Autodesk Fusion 360 part; units mm, degrees
(part 3 of 3)
  line L1749 (208.3944, 281.0774) -> (206.5826, 280.7265)
  line L1750 (222.9841, 283.0826) -> (221.6889, 282.9561)
  line L1751 (248.9543, 186.6306) -> (249.0021, 186.3543)
  line L1752 (195.2165, 277.6676) -> (195.1345, 277.5743)
  line L1753 (282.2262, 282.3149) -> (280.3205, 282.5523)
  line L1754 (274.0771, 283.1906) -> (271.0467, 283.4676)
  line L1755 (195.1011, 277.4923) -> (198.2479, 273.2051)
  line L1756 (284.0442, 282.0682) -> (282.2262, 282.3149)
  line L1757 (206.5826, 280.7265) -> (204.8864, 280.373)
  line L1758 (212.3645, 281.7592) -> (210.3217, 281.4227)
  line L1759 (195.3395, 277.767) -> (195.2165, 277.6676)
  line L1760 (229.8917, 283.6109) -> (228.4526, 283.5204)
  line L1761 (249.0554, 186.0895) -> (249.1147, 185.8662)
  line L1762 (249.0021, 186.3543) -> (249.0554, 186.0895)
  line L1763 (276.246, 282.992) -> (274.0771, 283.1906)
  line L1764 (291.8211, 280.761) -> (290.4407, 281.0262)
  line L1765 (297.4131, 279.4996) -> (296.4692, 279.7372)
  line L1766 (299.3168, 278.9841) -> (298.2698, 279.2731)
  line L1767 (195.1345, 277.5743) -> (195.1112, 277.5316)
  line L1768 (221.6889, 282.9561) -> (220.4225, 282.8236)
  line L1769 (274.6565, 267.6572) -> (275.3635, 267.5207)
  line L1770 (291.1421, 264.0873) -> (291.6993, 264.4176)
  line L1771 (264.1428, 259.2261) -> (264.6603, 261.8646)
  line L1772 (284.4844, 260.9375) -> (284.5965, 260.9561)
  line L1773 (266.1501, 268.214) -> (266.1932, 268.2563)
  line L1774 (279.5002, 266.3305) -> (280.0419, 266.1024)
  line L1775 (278.9516, 266.543) -> (279.5002, 266.3305)
  line L1776 (248.8733, 187.0975) -> (248.9543, 186.6306)
  line L1777 (281.7836, 265.2546) -> (283.7059, 263.1269)
  line L1778 (266.0031, 267.9084) -> (266.0551, 268.04)
  line L1779 (249.2535, 185.6642) -> (249.2927, 185.6866)
  line L1780 (285.7031, 261.3881) -> (286.7992, 261.8821)
  line L1781 (249.1147, 185.8662) -> (249.1468, 185.7794)
  line L1782 (249.2161, 185.6747) -> (249.2345, 185.6656)
  line L1783 (280.8861, 265.7216) -> (281.1981, 265.5867)
  line L1784 (266.1041, 268.1418) -> (266.1501, 268.214)
  line L1785 (277.2718, 267.0843) -> (277.8367, 266.9201)
  line L1786 (280.5762, 265.859) -> (280.8861, 265.7216)
  line L1787 (266.0551, 268.04) -> (266.1041, 268.1418)
  line L1788 (284.3283, 260.9546) -> (284.3773, 260.9402)
  line L1789 (272.8993, 267.9499) -> (273.424, 267.8705)
  line L1790 (272.4361, 268.0131) -> (272.8993, 267.9499)
  line L1791 (265.762, 267.0883) -> (265.8894, 267.557)
  line L1792 (290.0115, 263.4568) -> (290.5793, 263.7671)
  line L1793 (290.5793, 263.7671) -> (291.1421, 264.0873)
  line L1794 (288.8641, 262.8646) -> (289.4395, 263.1561)
  line L1795 (265.4627, 265.8028) -> (265.6201, 266.5033)
  line L1796 (265.6201, 266.5033) -> (265.762, 267.0883)
  line L1797 (249.1806, 185.7144) -> (249.2161, 185.6747)
  line L1798 (284.2839, 260.9802) -> (284.3283, 260.9546)
  line L1799 (284.8032, 261.0126) -> (285.003, 261.0906)
  line L1800 (283.7059, 263.1269) -> (284.2839, 260.9802)
  line L1801 (281.3514, 265.5148) -> (281.501, 265.4369)
  line L1802 (265.0979, 264.0592) -> (265.4627, 265.8028)
  line L1803 (249.3339, 185.7457) -> (258.622, 231.7438)
  line L1804 (281.1981, 265.5867) -> (281.3514, 265.5148)
  line L1805 (249.2345, 185.6656) -> (249.2535, 185.6642)
  line L1806 (288.2859, 262.5822) -> (288.8641, 262.8646)
  line L1807 (281.6455, 265.3509) -> (281.7836, 265.2546)
  line L1808 (265.8894, 267.557) -> (266.0031, 267.9084)
  line L1809 (289.4395, 263.1561) -> (290.0115, 263.4568)
  line L1810 (275.3635, 267.5207) -> (276.1304, 267.3625)
  line L1811 (278.3969, 266.7396) -> (278.9516, 266.543)
  line L1812 (262.8388, 252.6458) -> (264.1428, 259.2261)
  line L1813 (284.7044, 260.9802) -> (284.8032, 261.0126)
  line L1814 (276.7028, 267.2318) -> (277.2718, 267.0843)
  line L1815 (274.0099, 267.7734) -> (274.6565, 267.6572)
  line L1816 (277.8367, 266.9201) -> (278.3969, 266.7396)
  line L1817 (273.424, 267.8705) -> (274.0099, 267.7734)
  line L1818 (284.5965, 260.9561) -> (284.7044, 260.9802)
  line L1819 (285.003, 261.0906) -> (285.7031, 261.3881)
  line L1820 (266.1932, 268.2563) -> (271.6958, 268.0958)
  line L1821 (291.6993, 264.4176) -> (292.2502, 264.7585)
  line L1822 (264.6603, 261.8646) -> (265.0979, 264.0592)
  line L1823 (280.0419, 266.1024) -> (280.5762, 265.859)
  line L1824 (284.3773, 260.9402) -> (284.4844, 260.9375)
  line L1825 (271.6958, 268.0958) -> (272.4361, 268.0131)
  line L1826 (258.622, 231.7438) -> (262.8388, 252.6458)
  line L1827 (292.2502, 264.7585) -> (292.7939, 265.11)
  line L1828 (286.7992, 261.8821) -> (288.2859, 262.5822)
  line L1829 (292.7939, 265.11) -> (293.3298, 265.4726)
  line L1830 (249.2927, 185.6866) -> (249.3339, 185.7457)
  line L1831 (276.1304, 267.3625) -> (276.7028, 267.2318)
  line L1832 (281.501, 265.4369) -> (281.6455, 265.3509)
  line L1833 (296.8008, 268.3446) -> (297.5669, 269.108)
  line L1834 (256.4399, 274.4982) -> (255.4396, 274.4952)
  line L1835 (294.8833, 266.6296) -> (295.3806, 267.0393)
  line L1836 (294.1268, 270.7552) -> (293.2879, 270.975)
  line L1837 (225.7816, 274.1169) -> (224.6982, 274.023)
  line L1838 (294.7936, 270.5692) -> (294.1268, 270.7552)
  line L1839 (255.1595, 274.4828) -> (255.0748, 274.4732)
  line L1840 (223.4692, 273.9056) -> (222.0948, 273.7634)
  line L1841 (293.2879, 270.975) -> (292.2757, 271.2235)
  line L1842 (295.7733, 270.2687) -> (295.2895, 270.4226)
  line L1843 (247.0886, 270.1383) -> (246.1685, 271.255)
  line L1844 (297.7654, 269.3164) -> (297.8145, 269.3775)
  line L1845 (276.8823, 273.6786) -> (275.0317, 273.8458)
  line L1846 (244.2152, 273.6532) -> (243.8236, 274.1236)
  line L1847 (243.4699, 274.5089) -> (243.4129, 274.5502)
  line L1848 (222.0948, 273.7634) -> (220.5752, 273.5951)
  line L1849 (291.089, 271.4951) -> (289.7268, 271.7846)
  line L1850 (284.2508, 272.7625) -> (282.4148, 273.0309)
  line L1851 (224.6982, 274.023) -> (223.4692, 273.9056)
  line L1852 (292.2757, 271.2235) -> (291.089, 271.4951)
  line L1853 (296.3401, 267.8965) -> (296.8008, 268.3446)
  line L1854 (246.1685, 271.255) -> (244.7346, 273.0159)
  line L1855 (275.0317, 273.8458) -> (273.1788, 273.9905)
  line L1856 (243.4129, 274.5502) -> (227.5104, 274.2394)
  line L1857 (249.1468, 185.7794) -> (249.1806, 185.7144)
  line L1858 (271.324, 274.1137) -> (269.4679, 274.2167)
  line L1859 (295.2895, 270.4226) -> (294.7936, 270.5692)
  line L1860 (322.7332, 314.692) -> (322.4298, 314.9296)
  line L1861 (323.7048, 313.8093) -> (323.3126, 314.1859)
  line L1862 (324.7886, 303.6366) -> (324.9042, 304.9171)
  line L1863 (310.0792, 323.0626) -> (308.9507, 323.6614)
  line L1864 (324.3257, 313.1815) -> (324.042, 313.474)
  line L1865 (297.9477, 328.7065) -> (296.4619, 329.2882)
  line L1866 (287.4008, 332.3961) -> (285.8705, 332.8536)
  line L1867 (320.2812, 316.2527) -> (320.1962, 316.3038)
  line L1868 (319.2981, 317.184) -> (318.947, 317.4895)
  line L1869 (324.9042, 304.9171) -> (324.9497, 305.5581)
  line L1870 (273.5972, 335.802) -> (271.5875, 336.1301)
  line L1871 (320.1155, 316.3616) -> (319.96, 316.5293)
  line L1872 (319.8006, 316.6988) -> (319.5813, 316.9188)
  line L1873 (224.4972, 335.6447) -> (223.0698, 335.3643)
  line L1874 (308.9507, 323.6614) -> (307.7593, 324.2748)
  line L1875 (259.2802, 337.7554) -> (258.6668, 337.7919)
  line L1876 (215.9614, 333.7319) -> (214.548, 333.3588)
  line L1877 (239.6725, 337.7845) -> (238.9752, 337.7305)
  line L1878 (228.8057, 336.401) -> (227.355, 336.1599)
  line L1879 (323.0278, 314.4444) -> (322.7332, 314.692)
  line L1880 (211.7322, 332.5656) -> (210.3306, 332.1453)
  line L1881 (302.3544, 326.8458) -> (300.8944, 327.4857)
  line L1882 (324.5868, 301.5321) -> (324.7886, 303.6366)
  line L1883 (210.3306, 332.1453) -> (208.9336, 331.7091)
  line L1884 (322.1188, 315.1576) -> (321.8012, 315.3769)
  line L1885 (316.2634, 319.4035) -> (315.5599, 319.859)
  line L1886 (319.96, 316.5293) -> (319.8006, 316.6988)
  line L1887 (320.8196, 315.9883) -> (320.642, 316.0799)
  line L1888 (323.3126, 314.1859) -> (323.0278, 314.4444)
  line L1889 (320.1962, 316.3038) -> (320.1155, 316.3616)
  line L1890 (313.9751, 320.843) -> (313.0927, 321.3687)
  line L1891 (318.0248, 318.2006) -> (317.4953, 318.5728)
  line L1892 (318.947, 317.4895) -> (318.5239, 317.83)
  line L1893 (315.5599, 319.859) -> (314.7973, 320.3393)
  line L1894 (320.4596, 316.1634) -> (320.2812, 316.2527)
  line L1895 (324.042, 313.474) -> (323.7048, 313.8093)
  line L1896 (321.4781, 315.588) -> (320.8196, 315.9883)
  line L1897 (314.7973, 320.3393) -> (313.9751, 320.843)
  line L1898 (217.378, 334.0893) -> (215.9614, 333.7319)
  line L1899 (299.4254, 328.1058) -> (297.9477, 328.7065)
  line L1900 (316.9084, 318.9743) -> (316.2634, 319.4035)
  line L1901 (322.4298, 314.9296) -> (322.1188, 315.1576)
  line L1902 (324.9795, 306.2) -> (324.9836, 312.4179)
  line L1903 (318.5239, 317.83) -> (318.0248, 318.2006)
  line L1904 (218.7976, 334.4312) -> (217.378, 334.0893)
  line L1905 (307.7593, 324.2748) -> (306.5046, 324.9014)
  line L1906 (324.9491, 312.4721) -> (324.8674, 312.5772)
  line L1907 (225.9257, 335.9099) -> (224.4972, 335.6447)
  line L1908 (214.548, 333.3588) -> (213.1381, 332.9701)
  line L1909 (293.4676, 330.3955) -> (291.96, 330.9219)
  line L1910 (276.8835, 335.1874) -> (276.1537, 335.3356)
  line L1911 (275.3627, 335.4875) -> (273.5972, 335.802)
  line L1912 (213.1381, 332.9701) -> (211.7322, 332.5656)
  line L1913 (324.8674, 312.5772) -> (324.5569, 312.9335)
  line L1914 (321.8012, 315.3769) -> (321.4781, 315.588)
  line L1915 (319.5813, 316.9188) -> (319.2981, 317.184)
  line L1916 (324.9497, 305.5581) -> (324.9795, 306.2)
  line L1917 (306.5046, 324.9014) -> (305.1859, 325.5398)
  line L1918 (313.0927, 321.3687) -> (312.1496, 321.9148)
  line L1919 (324.9836, 312.4179) -> (324.9491, 312.4721)
  line L1920 (320.642, 316.0799) -> (320.4596, 316.1634)
  line L1921 (324.5569, 312.9335) -> (324.3257, 313.1815)
  line L1922 (311.1453, 322.4799) -> (310.0792, 323.0626)
  line L1923 (258.6668, 337.7919) -> (240.0115, 337.8045)
  line L1924 (317.4953, 318.5728) -> (316.9084, 318.9743)
  line L1925 (305.1859, 325.5398) -> (303.8026, 326.1884)
  line L1926 (261.1143, 337.5583) -> (260.5038, 337.6319)
  line L1927 (282.7966, 333.72) -> (281.2539, 334.1295)
  line L1928 (276.1537, 335.3356) -> (275.3627, 335.4875)
  line L1929 (264.0969, 337.1857) -> (261.1143, 337.5583)
  line L1930 (237.9214, 337.6332) -> (236.5123, 337.4828)
  line L1931 (294.9684, 329.851) -> (293.4676, 330.3955)
  line L1932 (300.8944, 327.4857) -> (299.4254, 328.1058)
  line L1933 (278.1594, 334.9028) -> (277.5521, 335.0431)
  line L1934 (279.7081, 334.5236) -> (278.1594, 334.9028)
  line L1935 (288.9262, 331.9218) -> (287.4008, 332.3961)
  line L1936 (277.5521, 335.0431) -> (276.8835, 335.1874)
  line L1937 (240.0115, 337.8045) -> (239.6725, 337.7845)
  line L1938 (200.6691, 328.7549) -> (199.3146, 328.2058)
  line L1939 (177.1697, 315.6333) -> (176.7433, 315.3633)
  line L1940 (284.3356, 333.2948) -> (282.7966, 333.72)
  line L1941 (173.7111, 312.2406) -> (173.6926, 312.1123)
  line L1942 (266.837, 336.8229) -> (264.0969, 337.1857)
  line L1943 (227.355, 336.1599) -> (225.9257, 335.9099)
  line L1944 (312.1496, 321.9148) -> (311.1453, 322.4799)
  line L1945 (259.8925, 337.6999) -> (259.2802, 337.7554)
  line L1946 (199.3146, 328.2058) -> (197.9676, 327.6402)
  line L1947 (197.9676, 327.6402) -> (196.6284, 327.0581)
  line L1948 (269.3339, 336.4707) -> (266.837, 336.8229)
  line L1949 (271.5875, 336.1301) -> (269.3339, 336.4707)
  line L1950 (290.446, 331.4305) -> (288.9262, 331.9218)
  line L1951 (223.0698, 335.3643) -> (221.6438, 335.0687)
  line L1952 (181.7405, 319.0373) -> (180.9539, 318.5041)
  line L1953 (230.1694, 336.618) -> (228.8057, 336.401)
  line L1954 (260.5038, 337.6319) -> (259.8925, 337.6999)
  line L1955 (236.5123, 337.4828) -> (234.7496, 337.2699)
  line L1956 (177.8228, 316.0135) -> (177.6023, 315.892)
  line L1957 (175.565, 314.5732) -> (175.3879, 314.4285)
  line L1958 (234.7496, 337.2699) -> (233.7361, 337.1369)
  line L1959 (206.155, 330.7888) -> (204.7741, 330.3046)
  line L1960 (296.4619, 329.2882) -> (294.9684, 329.851)
  line L1961 (191.3572, 324.5639) -> (190.0625, 323.8985)
  line L1962 (202.0308, 329.2877) -> (200.6691, 328.7549)
  line L1963 (285.8705, 332.8536) -> (284.3356, 333.2948)
  line L1964 (233.7361, 337.1369) -> (232.6348, 336.9848)
  line L1965 (178.0471, 316.128) -> (177.8228, 316.0135)
  line L1966 (173.6724, 310.891) -> (173.687, 310.2069)
  line L1967 (220.2196, 334.7577) -> (218.7976, 334.4312)
  line L1968 (232.6348, 336.9848) -> (231.4459, 336.8122)
  line L1969 (221.6438, 335.0687) -> (220.2196, 334.7577)
  line L1970 (303.8026, 326.1884) -> (302.3544, 326.8458)
  line L1971 (175.2175, 314.2767) -> (175.0547, 314.1173)
  line L1972 (231.4459, 336.8122) -> (230.1694, 336.618)
  line L1973 (238.9752, 337.7305) -> (237.9214, 337.6332)
  line L1974 (203.3992, 329.8043) -> (202.0308, 329.2877)
  line L1975 (190.0625, 323.8985) -> (188.7779, 323.2162)
  line L1976 (175.9345, 314.8439) -> (175.7475, 314.7115)
  line L1977 (175.3879, 314.4285) -> (175.2175, 314.2767)
  line L1978 (291.96, 330.9219) -> (290.446, 331.4305)
  line L1979 (281.2539, 334.1295) -> (279.7081, 334.5236)
  line L1980 (178.3376, 316.3185) -> (178.1982, 316.2147)
extrude "Extrude1" add sketch "Tesla Shield" against normal blind 1 contours L0 L4 L5 L6 L7 L8 L9 L10 L12 L13 L14 L17 L19 L20 L21 L22 L23 L24 L25 L27 L28 L29 L30 L33 L34 L35 L36 L37 L39 L40 L41 L43 L44 L45 L47 L48 L49 L51 L52 L60 L61 L64 L65 L66 L67 L68 L69 L70 L71 L72 L73 L74 L75 L76 L77 L78 L79 L80 L81 L82 L83 L84 L85 L86 L87 L88 L89 L90 L91 L92 L93 L94 L95 L96 L97 L98 L99 L1195 L1196 L1204 L1208 L1210 L1220 L1236 L1237 L1238 L1239 L1240 L1241 L1242 L1243 L1244 L1245 L1246 L1247 L1248 L1249 L1250 L1251 L1252 L1253 L1254 L1255 L1256 L1257 L1258 L1259 L1260 L1261 L1262 L1263 L1264 L1265 L1266 L1267 L1268 L1269 L1270 L1271 L1272 L1273 L1274 L1275 L1276 L1277 L1278 L1279 L1280 L1281 L1282 L1283 L1284 L1285 L1286 L1287 L1288 L1289 L1290 L1291 L1292 L1293 L1294 L1295 L1296 L1297 L1298 L1299 L1300 L1301 L1302 L1303 L1304 L1305 L1306 L1307 L1308 L1309 L1310 L1311 L1312 L1313 L1314 L1315 L1316 L1317 L1318 L1319 L1320 L1321 L1322 L1323 L1324 L1325 L1326 L1327 L1328 L1329 L1330 L1331 L1332 L1333 L1334 L1335 L1336 L1337 L1338 L1339 L1340 L1341 L1342 L1343 L1344 L1345 L1346 L1347 L1348 L1349 L1350 L1351 L1352 L1353 L1354 L1355 L1356 L1357 L1358 L1359 L1360 L1361 L1362 L1363 L1364 L1365 L1366 L1367 L1368 L1369 L1370 L1371 L1372 L1373 L1374 L1375 L1376 L1377 L1378 L1379 L1380 L1381 L1382 L1383 L1384 L1385 L1386 L1387 L1388 L1389 L1390 L1391 L1392 L1393 L1394 L1395 L1396 L1397 L1398 L1399 L1400 L1401 L1402 L1403 L1404 L1405 L1406 L1407 L1408 L1412 L1414 L1415 L1416 L1417 L1418 L1419 L1860 L1861 L1862 L1863 L1864 L1865 L1866 L1867 L1868 L1869 L1870 L1871 L1872 L1873 L1874 L1875 L1876 L1877 L1878 L1879 L1880 L1881 L1882 L1883 L1884 L1885 L1886 L1887 L1888 L1889 L1890 L1891 L1892 L1893 L1894 L1895 L1896 L1897 L1898 L1899 L1900 L1901 L1902 L1903 L1904 L1905 L1906 L1907 L1908 L1909 L1910 L1911 L1912 L1913 L1914 L1915 L1916 L1917 L1918 L1919 L1920 L1921 L1922 L1923 L1924 L1925 L1926 L1927 L1928 L1929 L1930 L1931 L1932 L1933 L1934 L1935 L1936 L1937 L1938 L1939 L1940 L1941 L1942 L1943 L1944 L1945 L1946 L1947 L1948 L1949 L1950 L1951 L1952 L1953 L1954 L1955 L1956 L1957 L1958 L1959 L1960 L1961 L1962 L1963 L1964 L1965 L1966 L1967 L1968 L1969 L1970 L1971 L1972 L1973 L1974 L1975 L1976 L1977 L1978 L1979 L1980 | L1 L2 L3 L11 L15 L16 L18 L26 L31 L32 L38 L42 L46 L50 L53 L54 L55 L56 L57 L58 L59 L62 L63 L927 L929 L931 L932 L934 L936 L937 L938 L940 L941 L944 L947 L963 L964 L968 L969 L970 L971 L972 L973 L974 L991 L993 L994 L995 L996 L997 L998 L999 L1000 L1001 L1002 L1003 L1004 L1005 L1006 L1007 L1008 L1009 L1010 L1011 L1013 L1014 L1015 L1016 L1017 L1018 L1019 L1020 L1021 L1022 L1023 L1024 L1025 L1026 L1027 L1028 L1029 L1030 L1031 L1032 L1033 L1034 L1035 L1037 L1038 L1039 L1040 L1042 L1043 L1044 L1045 L1046 L1047 L1048 L1049 L1050 L1051 L1052 L1053 L1054 L1055 L1056 L1057 L1058 L1059 L1060 L1061 L1062 L1063 L1064 L1065 L1066 L1067 L1068 L1069 L1070 L1071 L1072 L1073 L1074 L1075 L1076 L1077 L1078 L1079 L1080 L1081 L1082 L1083 L1084 L1085 L1086 L1087 L1088 L1089 L1090 L1091 L1092 L1093 L1094 L1095 L1096 L1097 L1098 L1099 L1100 L1101 L1102 L1103 L1104 L1105 L1106 L1107 L1108 L1109 L1110 L1111 L1112 L1113 L1114 L1115 L1116 L1117 L1118 L1119 L1120 L1121 L1122 L1123 L1124 L1125 L1126 L1127 L1128 L1129 L1130 L1131 L1132 L1133 L1134 L1135 L1136 L1137 L1138 L1139 L1140 L1141 L1142 L1143 L1144 L1145 L1146 L1147 L1148 L1149 L1150 L1151 L1152 L1153 L1154 L1155 L1156 L1157 L1158 L1159 L1160 L1161 L1162 L1163 L1164 L1165 L1166 L1167 L1168 L1169 L1170 L1171 L1172 L1173 L1174 L1175 L1176 L1177 L1178 L1179 L1180 L1181 L1182 L1183 L1184 L1185 L1186 L1187 L1188 L1189 L1190 L1191 L1192 L1193 L1194 L1197 L1198 L1199 L1200 L1201 L1202 L1203 L1205 L1206 L1207 L1209 L1211 L1212 L1213 L1214 L1215 L1216 L1217 L1218 L1219 L1221 L1222 L1223 L1224 L1225 L1226 L1227 L1228 L1229 L1230 L1231 L1232 L1233 L1234 L1235 | L100 L101 L102 L103 L104 L105 L106 L107 L108 L109 L110 L111 L112 L113 L114 L115 L116 L117 L118 L119 L120 L121 L122 L123 L124 L125 L126 L127 L128 L129 L130 L131 L132 L133 L134 L135 L136 L137 L138 L139 L140 L141 L142 L143 L144 L145 L146 L147 L148 L149 L150 L151 L152 L153 L154 L155 L156 L157 L158 L159 L160 L161 L162 L163 L165 L166 L167 L168 L169 L170 L171 L172 L173 L175 L177 L178 L179 L180 L181 L182 L183 L185 L186 L190 L191 L192 L193 L194 L195 L196 L197 L200 L201 L203 L205 L206 L207 L208 L209 L210 L211 L212 L214 L215 L217 L218 L219 L220 L221 L222 L223 L224 L225 L226 L227 L230 L232 L234 L241 L252 L253 L254 L259 L260 L272 L273 L274 L279 L281 L284 L286 L1751 L1761 L1762 L1769 L1770 L1771 L1772 L1773 L1774 L1775 L1776 L1777 L1778 L1779 L1780 L1781 L1782 L1783 L1784 L1785 L1786 L1787 L1788 L1789 L1790 L1791 L1792 L1793 L1794 L1795 L1796 L1797 L1798 L1799 L1800 L1801 L1802 L1803 L1804 L1805 L1806 L1807 L1808 L1809 L1810 L1811 L1812 L1813 L1814 L1815 L1816 L1817 L1818 L1819 L1820 L1821 L1822 L1823 L1824 L1825 L1826 L1827 L1828 L1829 L1830 L1831 L1832 L1833 L1834 L1835 L1836 L1837 L1838 L1839 L1840 L1841 L1842 L1843 L1844 L1845 L1846 L1847 L1848 L1849 L1850 L1851 L1852 L1853 L1854 L1855 L1856 L1857 L1858 L1859 | L164 L174 L176 L184 L187 L188 L189 L198 L199 L202 L204 L213 L216 L228 L229 L231 L233 L235 L236 L237 L238 L239 L240 L242 L243 L244 L245 L246 L247 L248 L249 L250 L251 L255 L256 L257 L258 L261 L262 L263 L264 L265 L266 L267 L268 L269 L270 L271 L275 L276 L277 L278 L280 L282 L283 L285 L287 L288 L289 L290 L291 L292 L293 L294 L295 L296 L297 L298 L299 L300 L301 L302 L303 L304 L305 L306 L307 L308 L309 L310 L311 L312 L313 L314 L315 L316 L317 L318 L319 L320 L321 L322 L323 L324 L325 L326 L327 L328 L329 L330 L331 L332 L333 L334 L335 L336 L337 L338 L339 L340 L341 L342 L343 L344 L345 L346 L347 L348 L349 L350 L351 L352 L353 L354 L355 L356 L357 L358 L359 L360 L361 L362 L363 L364 L365 L366 L367 L368 L369 L370 L371 L372 L373 L374 L375 L376 L377 L378 L379 L380 L381 L382 L383 L384 L385 L386 L387 L388 L389 L390 L391 L392 L393 L394 L395 L396 L397 L398 L399 L400 L401 L402 L403 L404 L405 L406 L407 L408 L409 L410 L411 L412 L413 L414 L415 L416 L417 L418 L419 L420 L421 L422 L423 L424 L425 L426 L427 L428 L429 L430 L431 L432 L433 L434 L435 L436 L437 L438 L439 L440 L441 L442 L443 L444 L445 L446 L447 L448 L449 L450 L451 L452 L453 L454 L455 L456 L457 L458 L459 L460 L461 L462 L463 L464 L465 L466 L467 L468 L469 L470 L471 L472 L473 L474 L475 L476 L477 L478 L479 L480 L481 L482 L483 L484 L485 L486 L487 L488 L489 L490 L491 L492 L493 L494 L495 L496 L497 L498 L499 L500 L501 L502 L503 L504 L505 L506 L507 L508 L509 L510 L511 L512 L513 L514 L515 L516 L517 L518 L519 L520 L521 L522 L523 L524 L525 L526 L527 L528 L529 L530 L531 L532 L533 L534 L535 L536 L537 L538 L539 L540 L541 L542 L543 L544 L545 L546 L547 L548 L549 L550 L551 L552 L553 L554 L555 L556 L557 L558 L559 L560 L561 L562 L563 L564 L565 L566 L567 L568 L569 L570 L571 L572 L573 L574 L575 L576 L577 L578 L579 L580 L581 L582 L583 L584 L585 L586 L587 L588 L589 L590 L591 L592 L593 L594 L595 L596 L597 L598 L599 L600 L601 L602 L603 L604 L605 L606 L607 L608 L609 L610 L611 L612 L613 L614 L615 L616 L618 L619 L620 L621 L622 L623 L624 L626 L627 L628 L629 L630 L631 L632 L633 L634 L635 L636 L637 L638 L639 L640 L641 L642 L643 L644 L645 L646 L650 L651 L652 L653 L654 L656 L657 L658 L659 L660 L661 L662 L663 L664 L665 L666 L667 L668 L670 L671 L672 L676 L683 L688 L689 L690 L692 L695 L700 L707 L712 L715 L719 L727 L732 L733 L735 | L617 L625 L647 L648 L649 L655 L669 L673 L674 L675 L677 L678 L679 L680 L681 L682 L684 L685 L686 L687 L691 L693 L694 L696 L697 L698 L699 L701 L702 L703 L704 L705 L706 L708 L709 L710 L711 L713 L714 L716 L717 L718 L720 L721 L722 L723 L724 L725 L726 L728 L729 L730 L731 L734 L736 L737 L738 L739 L740 L741 L742 L743 L744 L745 L746 L747 L748 L749 L750 L751 L752 L753 L754 L755 L756 L757 L758 L759 L760 L761 L762 L763 L764 L765 L766 L767 L768 L769 L770 L771 L772 L773 L774 L775 L776 L777 L778 L779 L780 L781 L782 L783 L784 L785 L786 L787 L788 L789 L790 L791 L792 L793 L794 L795 L796 L797 L798 L799 L800 L801 L802 L803 L804 L805 L806 L807 L808 L809 L810 L811 L812 L813 L814 L815 L816 L817 L818 L819 L820 L821 L822 L823 L824 L825 L826 L827 L828 L829 L830 L831 L832 L833 L834 L835 L836 L837 L838 L839 L840 L841 L842 L843 L844 L845 L846 L847 L848 L849 L850 L851 L852 L853 L854 L855 L856 L857 L858 L859 L860 L861 L862 L863 L864 L865 L866 L867 L868 L869 L870 L871 L872 L873 L874 L875 L876 L877 L878 L879 L880 L881 L882 L883 L884 L885 L886 L887 L888 L889 L890 L891 L892 L893 L894 L895 L896 L897 L898 L899 L900 L901 L902 L903 L904 L905 L906 L907 L908 L909 L910 L911 L912 L913 L914 L915 L916 L917 L918 L919 L920 L921 L922 L923 L924 L925 L926 L928 L930 L933 L935 L939 L942 L943 L945 L946 L948 L949 L950 L951 L952 L953 L954 L955 L956 L957 L958 L959 L960 L961 L962 L965 L966 L967 L975 L976 L977 L978 L979 L980 L981 L982 L983 L984 L985 L986 L987 L988 L989 L990 L992 L1012 L1036 L1041 | L1409 L1420 L1421 L1422 L1423 L1424 L1426 L1429 L1433 L1438 L1439 L1440 L1443 L1444 L1449 L1474 L1476 L1477 L1480 L1481 | L1410 L1411 L1413 L1425 L1427 L1428 L1430 L1431 L1432 L1434 L1435 L1436 L1437 L1441 L1442 L1445 L1446 L1447 L1448 L1450 L1451 L1452 L1454 L1455 L1461 L1462 L1463 L1464 L1465 L1466 L1467 L1470 L1472 L1473 L1475 L1478 L1483 L1485 L1488 L1490 L1492 L1494 L1498 L1500 L1501 L1505 L1507 L1514 L1535 | L1453 L1456 L1457 L1458 L1468 L1471 L1479 L1482 L1484 L1486 L1491 L1493 L1495 L1499 L1502 L1503 L1504 L1506 L1508 L1509 L1511 L1512 L1513 L1515 L1523 L1538 L1541 L1542 L1554 L1560 L1561 L1565 L1567 L1569 L1572 | L1459 L1460 L1469 L1487 L1489 L1496 L1497 L1510 L1573 | L1516 L1521 L1530 L1532 L1536 L1537 L1539 L1544 L1546 L1547 L1549 L1551 L1556 L1558 L1559 L1562 L1566 L1568 L1577 L1578 | L1517 L1519 L1520 L1522 L1524 L1526 L1527 L1528 L1529 L1534 L1540 L1543 L1548 L1550 L1553 L1557 L1563 L1564 L1570 L1571 L1575 L1576 L1579 | L1518 L1525 L1531 L1533 L1545 L1552 L1555 L1574 L1581 L1585 L1599 L1600 L1605 L1607 L1610 L1613 L1617 L1626 L1637 L1639 | L1580 L1586 L1588 L1589 L1592 L1593 L1594 L1595 L1596 L1598 L1601 L1603 L1608 L1609 L1611 L1612 L1619 L1620 L1621 L1624 L1628 L1629 L1630 L1632 L1633 L1641 L1642 L1643 L1644 L1645 L1646 L1647 L1648 L1649 L1650 L1651 L1652 L1653 L1654 L1655 L1656 L1657 L1658 L1659 L1660 L1661 L1662 L1663 L1664 L1665 L1666 L1667 L1668 L1669 L1670 L1672 L1673 L1674 L1675 L1676 L1677 L1678 L1679 L1680 L1681 L1682 L1683 L1684 L1685 L1686 L1687 L1688 L1689 L1690 L1691 L1692 L1694 L1695 L1696 L1697 L1698 L1699 L1700 L1701 L1702 L1703 L1704 L1705 L1706 L1707 L1708 L1709 L1710 L1711 L1712 L1713 L1714 L1715 L1716 L1717 L1718 L1719 L1720 L1721 L1722 L1723 L1724 L1725 L1726 L1727 L1728 L1729 L1730 L1731 L1732 L1733 L1734 L1735 L1736 L1737 L1738 L1739 L1740 L1741 L1742 L1743 L1744 L1745 L1746 L1747 L1748 L1749 L1750 L1752 L1753 L1754 L1755 L1756 L1757 L1758 L1759 L1760 L1763 L1764 L1765 L1766 L1767 L1768 | L1582 L1583 L1584 L1587 L1590 L1591 L1597 L1602 L1604 L1606 L1614 L1615 L1616 L1618 L1622 L1623 L1625 L1627 L1631 L1634 L1635 L1636 L1638 L1640 L1671 L1693 makes body 1
extrude "Extrude2" add sketch "Tesla Shield" along normal blind 2 bodies 1
extrude "Extrude3" add sketch "Tesla Shield" along normal blind 2 separate body contours L100 L101 L102 L103 L104 L105 L106 L107 L108 L109 L110 L111 L112 L113 L114 L115 L116 L117 L118 L119 L120 L121 L122 L123 L124 L125 L126 L127 L128 L129 L130 L131 L132 L133 L134 L135 L136 L137 L138 L139 L140 L141 L142 L143 L144 L145 L146 L147 L148 L149 L150 L151 L152 L153 L154 L155 L156 L157 L158 L159 L160 L161 L162 L163 L165 L166 L167 L168 L169 L170 L171 L172 L173 L175 L177 L178 L179 L180 L181 L182 L183 L185 L186 L190 L191 L192 L193 L194 L195 L196 L197 L200 L201 L203 L205 L206 L207 L208 L209 L210 L211 L212 L214 L215 L217 L218 L219 L220 L221 L222 L223 L224 L225 L226 L227 L230 L232 L234 L241 L252 L253 L254 L259 L260 L272 L273 L274 L279 L281 L284 L286 L1751 L1761 L1762 L1769 L1770 L1771 L1772 L1773 L1774 L1775 L1776 L1777 L1778 L1779 L1780 L1781 L1782 L1783 L1784 L1785 L1786 L1787 L1788 L1789 L1790 L1791 L1792 L1793 L1794 L1795 L1796 L1797 L1798 L1799 L1800 L1801 L1802 L1803 L1804 L1805 L1806 L1807 L1808 L1809 L1810 L1811 L1812 L1813 L1814 L1815 L1816 L1817 L1818 L1819 L1820 L1821 L1822 L1823 L1824 L1825 L1826 L1827 L1828 L1829 L1830 L1831 L1832 L1833 L1834 L1835 L1836 L1837 L1838 L1839 L1840 L1841 L1842 L1843 L1844 L1845 L1846 L1847 L1848 L1849 L1850 L1851 L1852 L1853 L1854 L1855 L1856 L1857 L1858 L1859 | L164 L174 L176 L184 L187 L188 L189 L198 L199 L202 L204 L213 L216 L228 L229 L231 L233 L235 L236 L237 L238 L239 L240 L242 L243 L244 L245 L246 L247 L248 L249 L250 L251 L255 L256 L257 L258 L261 L262 L263 L264 L265 L266 L267 L268 L269 L270 L271 L275 L276 L277 L278 L280 L282 L283 L285 L287 L288 L289 L290 L291 L292 L293 L294 L295 L296 L297 L298 L299 L300 L301 L302 L303 L304 L305 L306 L307 L308 L309 L310 L311 L312 L313 L314 L315 L316 L317 L318 L319 L320 L321 L322 L323 L324 L325 L326 L327 L328 L329 L330 L331 L332 L333 L334 L335 L336 L337 L338 L339 L340 L341 L342 L343 L344 L345 L346 L347 L348 L349 L350 L351 L352 L353 L354 L355 L356 L357 L358 L359 L360 L361 L362 L363 L364 L365 L366 L367 L368 L369 L370 L371 L372 L373 L374 L375 L376 L377 L378 L379 L380 L381 L382 L383 L384 L385 L386 L387 L388 L389 L390 L391 L392 L393 L394 L395 L396 L397 L398 L399 L400 L401 L402 L403 L404 L405 L406 L407 L408 L409 L410 L411 L412 L413 L414 L415 L416 L417 L418 L419 L420 L421 L422 L423 L424 L425 L426 L427 L428 L429 L430 L431 L432 L433 L434 L435 L436 L437 L438 L439 L440 L441 L442 L443 L444 L445 L446 L447 L448 L449 L450 L451 L452 L453 L454 L455 L456 L457 L458 L459 L460 L461 L462 L463 L464 L465 L466 L467 L468 L469 L470 L471 L472 L473 L474 L475 L476 L477 L478 L479 L480 L481 L482 L483 L484 L485 L486 L487 L488 L489 L490 L491 L492 L493 L494 L495 L496 L497 L498 L499 L500 L501 L502 L503 L504 L505 L506 L507 L508 L509 L510 L511 L512 L513 L514 L515 L516 L517 L518 L519 L520 L521 L522 L523 L524 L525 L526 L527 L528 L529 L530 L531 L532 L533 L534 L535 L536 L537 L538 L539 L540 L541 L542 L543 L544 L545 L546 L547 L548 L549 L550 L551 L552 L553 L554 L555 L556 L557 L558 L559 L560 L561 L562 L563 L564 L565 L566 L567 L568 L569 L570 L571 L572 L573 L574 L575 L576 L577 L578 L579 L580 L581 L582 L583 L584 L585 L586 L587 L588 L589 L590 L591 L592 L593 L594 L595 L596 L597 L598 L599 L600 L601 L602 L603 L604 L605 L606 L607 L608 L609 L610 L611 L612 L613 L614 L615 L616 L618 L619 L620 L621 L622 L623 L624 L626 L627 L628 L629 L630 L631 L632 L633 L634 L635 L636 L637 L638 L639 L640 L641 L642 L643 L644 L645 L646 L650 L651 L652 L653 L654 L656 L657 L658 L659 L660 L661 L662 L663 L664 L665 L666 L667 L668 L670 L671 L672 L676 L683 L688 L689 L690 L692 L695 L700 L707 L712 L715 L719 L727 L732 L733 L735 | L617 L625 L647 L648 L649 L655 L669 L673 L674 L675 L677 L678 L679 L680 L681 L682 L684 L685 L686 L687 L691 L693 L694 L696 L697 L698 L699 L701 L702 L703 L704 L705 L706 L708 L709 L710 L711 L713 L714 L716 L717 L718 L720 L721 L722 L723 L724 L725 L726 L728 L729 L730 L731 L734 L736 L737 L738 L739 L740 L741 L742 L743 L744 L745 L746 L747 L748 L749 L750 L751 L752 L753 L754 L755 L756 L757 L758 L759 L760 L761 L762 L763 L764 L765 L766 L767 L768 L769 L770 L771 L772 L773 L774 L775 L776 L777 L778 L779 L780 L781 L782 L783 L784 L785 L786 L787 L788 L789 L790 L791 L792 L793 L794 L795 L796 L797 L798 L799 L800 L801 L802 L803 L804 L805 L806 L807 L808 L809 L810 L811 L812 L813 L814 L815 L816 L817 L818 L819 L820 L821 L822 L823 L824 L825 L826 L827 L828 L829 L830 L831 L832 L833 L834 L835 L836 L837 L838 L839 L840 L841 L842 L843 L844 L845 L846 L847 L848 L849 L850 L851 L852 L853 L854 L855 L856 L857 L858 L859 L860 L861 L862 L863 L864 L865 L866 L867 L868 L869 L870 L871 L872 L873 L874 L875 L876 L877 L878 L879 L880 L881 L882 L883 L884 L885 L886 L887 L888 L889 L890 L891 L892 L893 L894 L895 L896 L897 L898 L899 L900 L901 L902 L903 L904 L905 L906 L907 L908 L909 L910 L911 L912 L913 L914 L915 L916 L917 L918 L919 L920 L921 L922 L923 L924 L925 L926 L928 L930 L933 L935 L939 L942 L943 L945 L946 L948 L949 L950 L951 L952 L953 L954 L955 L956 L957 L958 L959 L960 L961 L962 L965 L966 L967 L975 L976 L977 L978 L979 L980 L981 L982 L983 L984 L985 L986 L987 L988 L989 L990 L992 L1012 L1036 L1041 | L1409 L1420 L1421 L1422 L1423 L1424 L1426 L1429 L1433 L1438 L1439 L1440 L1443 L1444 L1449 L1474 L1476 L1477 L1480 L1481 | L1410 L1411 L1413 L1425 L1427 L1428 L1430 L1431 L1432 L1434 L1435 L1436 L1437 L1441 L1442 L1445 L1446 L1447 L1448 L1450 L1451 L1452 L1454 L1455 L1461 L1462 L1463 L1464 L1465 L1466 L1467 L1470 L1472 L1473 L1475 L1478 L1483 L1485 L1488 L1490 L1492 L1494 L1498 L1500 L1501 L1505 L1507 L1514 L1535 | L1453 L1456 L1457 L1458 L1468 L1471 L1479 L1482 L1484 L1486 L1491 L1493 L1495 L1499 L1502 L1503 L1504 L1506 L1508 L1509 L1511 L1512 L1513 L1515 L1523 L1538 L1541 L1542 L1554 L1560 L1561 L1565 L1567 L1569 L1572 | L1459 L1460 L1469 L1487 L1489 L1496 L1497 L1510 L1573 | L1516 L1521 L1530 L1532 L1536 L1537 L1539 L1544 L1546 L1547 L1549 L1551 L1556 L1558 L1559 L1562 L1566 L1568 L1577 L1578 | L1517 L1519 L1520 L1522 L1524 L1526 L1527 L1528 L1529 L1534 L1540 L1543 L1548 L1550 L1553 L1557 L1563 L1564 L1570 L1571 L1575 L1576 L1579 | L1518 L1525 L1531 L1533 L1545 L1552 L1555 L1574 L1581 L1585 L1599 L1600 L1605 L1607 L1610 L1613 L1617 L1626 L1637 L1639 | L1580 L1586 L1588 L1589 L1592 L1593 L1594 L1595 L1596 L1598 L1601 L1603 L1608 L1609 L1611 L1612 L1619 L1620 L1621 L1624 L1628 L1629 L1630 L1632 L1633 L1641 L1642 L1643 L1644 L1645 L1646 L1647 L1648 L1649 L1650 L1651 L1652 L1653 L1654 L1655 L1656 L1657 L1658 L1659 L1660 L1661 L1662 L1663 L1664 L1665 L1666 L1667 L1668 L1669 L1670 L1672 L1673 L1674 L1675 L1676 L1677 L1678 L1679 L1680 L1681 L1682 L1683 L1684 L1685 L1686 L1687 L1688 L1689 L1690 L1691 L1692 L1694 L1695 L1696 L1697 L1698 L1699 L1700 L1701 L1702 L1703 L1704 L1705 L1706 L1707 L1708 L1709 L1710 L1711 L1712 L1713 L1714 L1715 L1716 L1717 L1718 L1719 L1720 L1721 L1722 L1723 L1724 L1725 L1726 L1727 L1728 L1729 L1730 L1731 L1732 L1733 L1734 L1735 L1736 L1737 L1738 L1739 L1740 L1741 L1742 L1743 L1744 L1745 L1746 L1747 L1748 L1749 L1750 L1752 L1753 L1754 L1755 L1756 L1757 L1758 L1759 L1760 L1763 L1764 L1765 L1766 L1767 L1768 | L1582 L1583 L1584 L1587 L1590 L1591 L1597 L1602 L1604 L1606 L1614 L1615 L1616 L1618 L1622 L1623 L1625 L1627 L1631 L1634 L1635 L1636 L1638 L1640 L1671 L1693 makes body 2 at (226.483, 300.392, 0) makes body 3 at (300.4215, 306.2061, 0) makes body 4 at (252.3435, 332.1295, 0) makes body 5 at (245.6899, 247.8361, 0) makes body 6 at (267.1103, 298.2424, 0) makes body 7 at (226.4369, 306.2086, 0) makes body 8 at (226.5711, 294.2972, 0) makes body 9 at (296.4963, 300.3978, 0) makes body 10 at (270.02, 188.1005, 0) makes body 11 at (250.2032, 281.1208, 0) makes body 12 at (247.6095, 306.2213, 0) makes body 13 at (198.7149, 306.224, 0)
